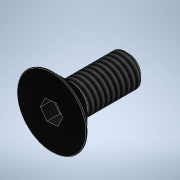
# Autodesk Inventor part: SCREW, FLAT HD, P, 5, M5X0_8X12MM
Saved by Autodesk Inventor 2022.4 (Build 264492000, 492)
## iProperties
Manager: 100-43730
Category: _
Created: 2001-02-21
Part Number: SCREW, FLAT HD, P, 5, M5X0_8X12MM
Material: Generic
Document SubType Name: Modeling
Designer: cdotson
Description: SCREW, FLAT HD, P, 5, M5X0_8X12MM
Checked By: 1UWXP
User Status: Released
Engr Approved By: P
Mfg Approved By: Clint.Matte
Density: 1 g/cm^3
Appearance: Glossy - Black
Mass: 0.324446 g
Surface Area: 3.76739 cm^2
Volume: 0.324446 cm^3
Control State: 0
Master: False
Checked Out: False
Shininess: 64.0
Length Units: 11269
Angle Units: 11279
Time Units: 11290
Mass Units: 11283
Length Display Precision: 3
Angle Display Precision: 2
CN_SERVICEABLE: _
CN_MASS: 0.000324
CL_runCount: 1
FinishProperty: ToBeSet
FIRST_DESCRIPTION: SCREW, FLAT HD, P, 5, M5X0_8X12MM
SECOND_DESCRIPTION: _
THIRD_DESCRIPTION: _
CN_DETAILER: -
CN_MFG_PART_NUM: _
CN_MFG_NAME: DEFAULT
STANDARDCLASSFLAG: P
CUSTOMERNUMBER: _
CN_DESIGNER: Clint.Matte
PTC_WM_ITERATION: 3
PTC_WM_ORGANIZATION_ID: CLWC
PTC_WM_LIFECYCLE: CLWC_CAD_LC
Density: 0.0
Volumn: 0.0
Area: 0.0
PropertySet Name: Model Information
Title: SCREW, FLAT HD, P, 5, M5X0_8X12MM_1UWXP.ipt
Subject: _
Author: -
Keywords: DEFAULT
Revision Number: 1
Autodesk Inventor part; units mm, degrees
ref_plane "YZ Plane" through (0, 0, 0) normal (1, 0, 0) x (0, 1, 0)
ref_plane "XZ Plane" through (0, 0, 0) normal (0, 1, 0) x (-1, 0, 0)
ref_plane "XY Plane" through (0, 0, 0) normal (0, 0, 1) x (1, 0, 0)
sketch "Sketch1" plane through (0, 0, 0) normal (0, 0, 1) x (1, 0, 0)
  circle A0 centre (0, 0) radius 2.5
  dimension "Diameter" = 5
  constraints: 1 centre point
  measures "Diameter" diameter of A0
extrude "Extrusion1" add sketch "Sketch1" along normal blind 8.9
sketch "Sketch2" plane through (0, 0, 8.9) normal (0, 0, 1) x (1, 0, 0)
  circle A0 centre (0, 0) radius 2.5 projected
extrude "Extrusion2" add sketch "Sketch2" along normal blind 3.1 draft 45
sketch "Sketch3" plane through (0, 0, 12) normal (0, 0, 1) x (1, 0, 0)
  circle A0 centre (0, 0) radius 5.6 projected
  circle A1 centre (0, 0) radius 1.7321 construction
  line L0 (0.725, 1.573) -> (1.7248, 0.1586)
  line L1 (1.7248, 0.1586) -> (0.9997, -1.4144)
  line L2 (0.9997, -1.4144) -> (-0.725, -1.573)
  line L3 (-0.725, -1.573) -> (-1.7248, -0.1586)
  line L4 (-1.7248, -0.1586) -> (-0.9997, 1.4144)
  line L5 (-0.9997, 1.4144) -> (0.725, 1.573)
  dimension "Hex_Width" = 3
  constraints: 12 end point, 6 point on circle, 4 equal length, 1 centre point, 1 coincident
  measures "Hex_Width" distance between parallel lines of L0 L3
extrude "Extrusion3" cut sketch "Sketch3" against normal blind 2 contours L0 L1 L2 L3 L4 L5
thread "Thread1" size "M5x0.8" class "4g6g" standard "ANSI Metric M Profile" length 8.9
chamfer "Chamfer2" distance 0.5 angle 45 1 edges at (-2.5, 0, 0)
fillet "Fillet1" radius 0.1 1 edges at (-5.6, 0, 12)
equation "\"d10\" = Thread_Length"
equation "\"d13\" = Chamfer"
equation "\"Thread_Length\" = 8.9"
equation "\"Length\" = 12"
equation "\"Chamfer\" = 0.5"
body "Solid1"
